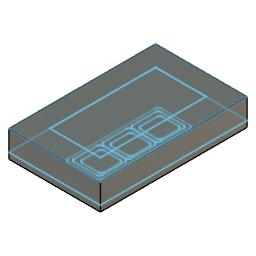
Hackpad (Autodesk Fusion 360 design; units mm, degrees)
part number: 2026-05-27-11-06-18-475
Autodesk Fusion 360 part; units mm, degrees
sketch "Sketch3" plane through (0, 0, 0) normal (0, 1, 0) x (1, 0, 0)
  line L0 (-10, 3.38, 10) -> (14.69, 3.38, 10)
  line L1 (14.69, 3.38, 10) -> (14.69, 3.38, 61.62)
  line L2 (14.69, 3.38, 61.62) -> (-10, 3.38, 61.62)
  line L3 (-10, 3.38, 61.62) -> (-10, 3.38, 10)
  line L4 (-20, 3.38) -> (24.69, 3.38)
  line L5 (24.69, 3.38, 0) -> (24.69, 3.38, 71.62)
  line L6 (24.69, 3.38, 71.62) -> (-20, 3.38, 71.62)
  line L7 (-20, 3.38, 71.62) -> (-20, 3.38, 0)
extrude "Extrude5" add sketch "Sketch3" along normal blind 3 contours L0 L1 L2 L3 in plane through (0, 0, -3.38) normal (0, 0, -1)
extrude "Extrude6" add sketch "Sketch3" along normal blind 10 contours L4 L5 L6 L7 in plane through (0, 0, -3.38) normal (0, 0, -1)
sketch "Sketch5" plane through (0, 0, -13.38) normal (0, 0, -1) x (1, 0, 0)
  line L0 (14.69, -61.62) -> (-10, -61.62)
  line L1 (-10, -61.62) -> (-10, -10)
  line L2 (-10, -10) -> (14.69, -10)
  line L3 (14.69, -10) -> (14.69, -61.62)
  line L4 (-20, -71.62) -> (24.69, -71.62)
  line L5 (24.69, -71.62) -> (24.69, 0)
  line L6 (24.69, 0) -> (-20, 0)
  line L7 (-20, 0) -> (-20, -71.62)
sketch "Sketch7" plane through (0, 0, -13.38) normal (0, 0, -1) x (1, 0, 0)
  line L0 (24.7, -71.6) -> (-20, -71.6)
  line L1 (-20, -71.6) -> (-20, 0)
  line L2 (-20, 0) -> (24.7, 0)
  line L3 (24.7, 0) -> (24.7, -71.6)
  constraint horizontal L0
  constraint vertical L1
  constraint horizontal L2
  constraint vertical L3
extrude "Extrude7" add sketch "Sketch5" along normal blind 3
sketch "keyboard-layout" plane through (0, 0, -16.38) normal (0, 0, -1) x (-1, 0, 0)
  line L0 (-7.433, 41.2046) -> (0.5045, 41.2046)
  line L1 (-8.733, 43.4219) -> (-9.1622, 43.7087)
  line L2 (-9.449, 44.1379) -> (-9.5497, 44.6442)
  line L3 (-8.2268, 43.3212) -> (-8.733, 43.4219)
  line L4 (-9.1622, 43.7087) -> (-9.449, 44.1379)
  line L5 (-8.6552, 40.3879) -> (-8.3685, 40.8171)
  line L6 (4.1079, 44.1379) -> (3.8212, 43.7087)
  line L7 (-8.2268, 43.3212) -> (-8.733, 43.4219)
  line L8 (-9.1622, 43.7087) -> (-9.449, 44.1379)
  line L9 (-8.7559, 46.2317) -> (-8.7559, 54.1691)
  line L10 (-8.7559, 54.1691) -> (-8.6552, 54.6754)
  line L11 (-8.3685, 55.1046) -> (-7.9393, 55.3914)
  line L12 (-9.449, 56.2629) -> (-9.1622, 56.6921)
  line L13 (1.7267, 45.7254) -> (1.4399, 45.2962)
  line L14 (3.8212, 56.6921) -> (4.1079, 56.2629)
  line L15 (3.392, 56.9789) -> (3.8212, 56.6921)
  line L16 (-7.9393, 45.0094) -> (-8.3685, 45.2962)
  line L17 (1.0107, 45.0094) -> (0.5045, 44.9087)
  line L18 (4.2086, 55.7566) -> (4.2086, 44.6442)
  line L19 (-7.433, 55.4921) -> (0.5045, 55.4921)
  line L20 (-8.3685, 55.1046) -> (-7.9393, 55.3914)
  line L21 (-8.7559, 46.2317) -> (-8.7559, 54.1691)
  line L22 (-9.1622, 56.6921) -> (-8.733, 56.9789)
  line L23 (-8.6552, 54.6754) -> (-8.3685, 55.1046)
  line L24 (0.5045, 55.4921) -> (1.0107, 55.3914)
  line L25 (-8.3685, 45.2962) -> (-8.6552, 45.7254)
  line L26 (-8.6552, 45.7254) -> (-8.7559, 46.2317)
  line L27 (2.8857, 43.3212) -> (-8.2268, 43.3212)
  line L28 (2.8857, 57.0796) -> (3.392, 56.9789)
  line L29 (0.5045, 55.4921) -> (1.0107, 55.3914)
  line L30 (1.0107, 55.3914) -> (1.4399, 55.1046)
  line L31 (-7.433, 44.9087) -> (-7.9393, 45.0094)
  line L32 (0.5045, 44.9087) -> (-7.433, 44.9087)
  line L33 (1.4399, 55.1046) -> (1.7267, 54.6754)
  line L34 (-8.733, 43.4219) -> (-9.1622, 43.7087)
  line L35 (-8.6552, 54.6754) -> (-8.3685, 55.1046)
  line L36 (1.8274, 54.1691) -> (1.8274, 46.2317)
  line L37 (3.8212, 43.7087) -> (3.392, 43.4219)
  line L38 (1.4399, 55.1046) -> (1.7267, 54.6754)
  line L39 (1.4399, 45.2962) -> (1.0107, 45.0094)
  line L40 (-9.449, 44.1379) -> (-9.5497, 44.6442)
  line L41 (1.7267, 54.6754) -> (1.8274, 54.1691)
  line L42 (1.8274, 54.1691) -> (1.8274, 46.2317)
  line L43 (1.4399, 45.2962) -> (1.0107, 45.0094)
  line L44 (-7.433, 55.4921) -> (0.5045, 55.4921)
  line L45 (0.5045, 44.9087) -> (-7.433, 44.9087)
  line L46 (-8.733, 56.9789) -> (-8.2268, 57.0796)
  line L47 (1.8274, 46.2317) -> (1.7267, 45.7254)
  line L48 (4.2086, 44.6442) -> (4.1079, 44.1379)
  line L49 (-7.9393, 55.3914) -> (-7.433, 55.4921)
  line L50 (4.1079, 56.2629) -> (4.2086, 55.7566)
  line L51 (-8.2268, 57.0796) -> (2.8857, 57.0796)
  line L52 (1.0107, 45.0094) -> (0.5045, 44.9087)
  line L53 (1.8274, 46.2317) -> (1.7267, 45.7254)
  line L54 (1.7267, 45.7254) -> (1.4399, 45.2962)
  line L55 (-7.433, 44.9087) -> (-7.9393, 45.0094)
  line L56 (-8.7559, 54.1691) -> (-8.6552, 54.6754)
  line L57 (-7.9393, 45.0094) -> (-8.3685, 45.2962)
  line L58 (1.0107, 55.3914) -> (1.4399, 55.1046)
  line L59 (-7.9393, 55.3914) -> (-7.433, 55.4921)
  line L60 (-8.3685, 45.2962) -> (-8.6552, 45.7254)
  line L61 (3.392, 43.4219) -> (2.8857, 43.3212)
  line L62 (-9.5497, 44.6442) -> (-9.5497, 55.7566)
  line L63 (-8.6552, 45.7254) -> (-8.7559, 46.2317)
  line L64 (1.7267, 54.6754) -> (1.8274, 54.1691)
  line L65 (2.8857, 42.7921) -> (3.392, 42.6914)
  line L66 (-8.6552, 17.1504) -> (-8.7559, 17.6567)
  line L67 (-7.9393, 26.8164) -> (-7.433, 26.9171)
  line L68 (2.8857, 42.7921) -> (3.392, 42.6914)
  line L69 (3.8212, 29.4212) -> (3.392, 29.1345)
  line L70 (-9.5497, 55.7566) -> (-9.449, 56.2629)
  line L71 (1.4399, 16.7212) -> (1.0107, 16.4345)
  line L72 (3.392, 29.1345) -> (2.8857, 29.0338)
  line L73 (-8.6552, 17.1504) -> (-8.7559, 17.6567)
  line L74 (-9.5497, 41.4692) -> (-9.449, 41.9754)
  line L75 (-7.433, 16.3338) -> (-7.9393, 16.4345)
  line L76 (0.5045, 16.3338) -> (-7.433, 16.3338)
  line L77 (1.8274, 17.6567) -> (1.7267, 17.1504)
  line L78 (-7.9393, 16.4345) -> (-8.3685, 16.7212)
  line L79 (-8.3685, 16.7212) -> (-8.6552, 17.1504)
  line L80 (-8.2268, 42.7921) -> (2.8857, 42.7921)
  line L81 (-7.9393, 16.4345) -> (-8.3685, 16.7212)
  line L82 (1.7267, 26.1004) -> (1.8274, 25.5942)
  line L83 (1.0107, 16.4345) -> (0.5045, 16.3338)
  line L84 (4.2086, 41.4692) -> (4.2086, 30.3567)
  line L85 (-9.1622, 29.4212) -> (-9.449, 29.8504)
  line L86 (-8.733, 42.6914) -> (-8.2268, 42.7921)
  line L87 (3.392, 42.6914) -> (3.8212, 42.4046)
  line L88 (4.1079, 29.8504) -> (3.8212, 29.4212)
  line L89 (-8.733, 29.1345) -> (-9.1622, 29.4212)
  line L90 (-8.2268, 42.7921) -> (2.8857, 42.7921)
  line L91 (1.8274, 25.5942) -> (1.8274, 17.6567)
  line L92 (4.1079, 29.8504) -> (3.8212, 29.4212)
  line L93 (-8.3685, 16.7212) -> (-8.6552, 17.1504)
  line L94 (-9.449, 29.8504) -> (-9.5497, 30.3567)
  line L95 (-9.5497, 41.4692) -> (-9.449, 41.9754)
  line L96 (4.2086, 41.4692) -> (4.2086, 30.3567)
  line L97 (4.2086, 30.3567) -> (4.1079, 29.8504)
  line L98 (4.1079, 41.9754) -> (4.2086, 41.4692)
  line L99 (0.5045, 26.9171) -> (1.0107, 26.8164)
  line L100 (3.8212, 42.4046) -> (4.1079, 41.9754)
  line L101 (4.2086, 30.3567) -> (4.1079, 29.8504)
  line L102 (1.4399, 26.5296) -> (1.7267, 26.1004)
  line L103 (-8.7559, 17.6567) -> (-8.7559, 25.5942)
  line L104 (2.8857, 29.0338) -> (-8.2268, 29.0338)
  line L105 (-9.5497, 30.3567) -> (-9.5497, 41.4692)
  line L106 (-9.1622, 42.4046) -> (-8.733, 42.6914)
  line L107 (-8.7559, 25.5942) -> (-8.6552, 26.1004)
  line L108 (-8.2268, 29.0338) -> (-8.733, 29.1345)
  line L109 (1.0107, 41.1039) -> (1.4399, 40.8171)
  line L110 (0.5045, 30.6213) -> (-7.433, 30.6213)
  line L111 (1.7267, 40.3879) -> (1.8274, 39.8817)
  line L112 (1.4399, 31.0087) -> (1.0107, 30.722)
  line L113 (-8.6552, 31.4379) -> (-8.7559, 31.9442)
  line L114 (0.5045, 41.2046) -> (1.0107, 41.1039)
  line L115 (-8.2268, 29.0338) -> (-8.733, 29.1345)
  line L116 (1.8274, 31.9442) -> (1.7267, 31.4379)
  line L117 (-8.3685, 40.8171) -> (-7.9393, 41.1039)
  line L118 (1.8274, 31.9442) -> (1.7267, 31.4379)
  line L119 (-7.9393, 41.1039) -> (-7.433, 41.2046)
  line L120 (1.7267, 40.3879) -> (1.8274, 39.8817)
  line L121 (-8.6552, 31.4379) -> (-8.7559, 31.9442)
  line L122 (-9.5497, 55.7566) -> (-9.449, 56.2629)
  line L123 (0.5045, 30.6213) -> (-7.433, 30.6213)
  line L124 (0.5045, 41.2046) -> (1.0107, 41.1039)
  line L125 (1.4399, 31.0087) -> (1.0107, 30.722)
  line L126 (1.0107, 30.722) -> (0.5045, 30.6213)
  line L127 (-7.433, 41.2046) -> (0.5045, 41.2046)
  line L128 (-7.433, 30.6213) -> (-7.9393, 30.722)
  line L129 (-8.7559, 39.8817) -> (-8.6552, 40.3879)
  line L130 (-8.7559, 39.8817) -> (-8.6552, 40.3879)
  line L131 (-8.7559, 31.9442) -> (-8.7559, 39.8817)
  line L132 (-7.9393, 41.1039) -> (-7.433, 41.2046)
  line L133 (1.8274, 39.8817) -> (1.8274, 31.9442)
  line L134 (-8.3685, 31.0087) -> (-8.6552, 31.4379)
  line L135 (-8.7559, 31.9442) -> (-8.7559, 39.8817)
  line L136 (-9.5497, 44.6442) -> (-9.5497, 55.7566)
  line L137 (-8.2268, 57.0796) -> (2.8857, 57.0796)
  line L138 (1.4399, 40.8171) -> (1.7267, 40.3879)
  line L139 (1.8274, 39.8817) -> (1.8274, 31.9442)
  line L140 (1.7267, 31.4379) -> (1.4399, 31.0087)
  line L141 (-8.733, 56.9789) -> (-8.2268, 57.0796)
  line L142 (2.8857, 57.0796) -> (3.392, 56.9789)
  line L143 (1.4399, 40.8171) -> (1.7267, 40.3879)
  line L144 (-9.1622, 56.6921) -> (-8.733, 56.9789)
  line L145 (-7.433, 30.6213) -> (-7.9393, 30.722)
  line L146 (3.392, 56.9789) -> (3.8212, 56.6921)
  line L147 (3.8212, 56.6921) -> (4.1079, 56.2629)
  line L148 (-7.9393, 30.722) -> (-8.3685, 31.0087)
  line L149 (-9.1622, 29.4212) -> (-9.449, 29.8504)
  line L150 (4.1079, 56.2629) -> (4.2086, 55.7566)
  line L151 (-8.6552, 40.3879) -> (-8.3685, 40.8171)
  line L152 (-8.3685, 31.0087) -> (-8.6552, 31.4379)
  line L153 (4.2086, 44.6442) -> (4.1079, 44.1379)
  line L154 (-9.449, 56.2629) -> (-9.1622, 56.6921)
  line L155 (3.392, 43.4219) -> (2.8857, 43.3212)
  line L156 (4.1079, 44.1379) -> (3.8212, 43.7087)
  line L157 (3.8212, 43.7087) -> (3.392, 43.4219)
  line L158 (2.8857, 43.3212) -> (-8.2268, 43.3212)
  line L159 (2.8857, 29.0338) -> (-8.2268, 29.0338)
  line L160 (1.0107, 41.1039) -> (1.4399, 40.8171)
  line L161 (1.0107, 30.722) -> (0.5045, 30.6213)
  line L162 (4.2086, 55.7566) -> (4.2086, 44.6442)
  line L163 (-11.1372, 14.7463) -> (-11.1372, 57.0795)
  line L164 (4.1079, 15.5629) -> (3.8212, 15.1337)
  line L165 (3.392, 14.847) -> (2.8857, 14.7463)
  line L166 (4.2086, 27.1817) -> (4.2086, 16.0692)
  line L167 (-11.0124, 57.6975) -> (-10.6722, 58.2021)
  line L168 (4.2086, 58.667) -> (4.8266, 58.5423)
  line L169 (-11.1372, 57.0795) -> (-11.0124, 57.6975)
  line L170 (-9.449, 29.8504) -> (-9.5497, 30.3567)
  line L171 (-7.9393, 30.722) -> (-8.3685, 31.0087)
  line L172 (-8.733, 29.1345) -> (-9.1622, 29.4212)
  line L173 (-10.1676, 58.5423) -> (-9.5497, 58.667)
  line L174 (-9.5497, 58.667) -> (4.2086, 58.667)
  line L175 (5.3312, 58.2021) -> (5.6714, 57.6975)
  line L176 (5.6714, 57.6975) -> (5.7961, 57.0795)
  line L177 (5.7961, 57.0795) -> (5.7961, 14.7463)
  line L178 (-10.6722, 13.6237) -> (-11.0163, 14.1388)
  line L179 (-8.3685, 40.8171) -> (-7.9393, 41.1039)
  line L180 (4.8266, 58.5423) -> (5.3312, 58.2021)
  line L181 (-10.6722, 58.2021) -> (-10.1676, 58.5423)
  line L182 (-9.5497, 13.1588) -> (-10.1572, 13.2796)
  line L183 (-8.2268, 28.5046) -> (2.8857, 28.5046)
  line L184 (2.8857, 28.5046) -> (3.392, 28.4039)
  line L185 (1.7267, 31.4379) -> (1.4399, 31.0087)
  line L186 (5.3312, 13.6237) -> (4.8162, 13.2796)
  line L187 (-9.1622, 28.1171) -> (-8.733, 28.4039)
  line L188 (-11.0163, 14.1388) -> (-11.1372, 14.7463)
  line L189 (-8.733, 28.4039) -> (-8.2268, 28.5046)
  line L190 (4.2086, 13.1588) -> (-9.5497, 13.1588)
  line L191 (3.392, 28.4039) -> (3.8212, 28.1171)
  line L192 (5.6753, 14.1388) -> (5.3312, 13.6237)
  line L193 (-8.2268, 14.7463) -> (-8.733, 14.847)
  line L194 (3.8212, 15.1337) -> (3.392, 14.847)
  line L195 (-9.5497, 16.0692) -> (-9.5497, 27.1817)
  line L196 (-10.1572, 13.2796) -> (-10.6722, 13.6237)
  line L197 (4.1079, 27.6879) -> (4.2086, 27.1817)
  line L198 (-9.449, 27.6879) -> (-9.1622, 28.1171)
  line L199 (-9.5497, 27.1817) -> (-9.449, 27.6879)
  line L200 (3.8212, 28.1171) -> (4.1079, 27.6879)
  line L201 (2.8857, 14.7463) -> (-8.2268, 14.7463)
  line L202 (5.7961, 14.7463) -> (5.6753, 14.1388)
  line L203 (4.8162, 13.2796) -> (4.2086, 13.1588)
  line L204 (4.2086, 16.0692) -> (4.1079, 15.5629)
  line L205 (-8.733, 14.847) -> (-9.1622, 15.1337)
  line L206 (-9.1622, 15.1337) -> (-9.449, 15.5629)
  line L207 (-9.449, 15.5629) -> (-9.5497, 16.0692)
  line L208 (-9.5497, 16.0692) -> (-9.5497, 27.1817)
  line L209 (-9.449, 27.6879) -> (-9.1622, 28.1171)
  line L210 (-9.5497, 27.1817) -> (-9.449, 27.6879)
  line L211 (-8.2268, 28.5046) -> (2.8857, 28.5046)
  line L212 (-9.1622, 28.1171) -> (-8.733, 28.4039)
  line L213 (-8.733, 28.4039) -> (-8.2268, 28.5046)
  line L214 (2.8857, 28.5046) -> (3.392, 28.4039)
  line L215 (3.392, 28.4039) -> (3.8212, 28.1171)
  line L216 (3.8212, 28.1171) -> (4.1079, 27.6879)
  line L217 (4.1079, 27.6879) -> (4.2086, 27.1817)
  line L218 (4.2086, 27.1817) -> (4.2086, 16.0692)
  line L219 (-8.2268, 14.7463) -> (-8.733, 14.847)
  line L220 (-9.449, 15.5629) -> (-9.5497, 16.0692)
  line L221 (4.1079, 15.5629) -> (3.8212, 15.1337)
  line L222 (-8.3685, 26.5296) -> (-7.9393, 26.8164)
  line L223 (1.4399, 26.5296) -> (1.7267, 26.1004)
  line L224 (-7.433, 16.3338) -> (-7.9393, 16.4345)
  line L225 (-7.433, 26.9171) -> (0.5045, 26.9171)
  line L226 (-8.733, 14.847) -> (-9.1622, 15.1337)
  line L227 (-7.9393, 26.8164) -> (-7.433, 26.9171)
  line L228 (-8.6552, 26.1004) -> (-8.3685, 26.5296)
  line L229 (1.7267, 26.1004) -> (1.8274, 25.5942)
  line L230 (-9.449, 41.9754) -> (-9.1622, 42.4046)
  line L231 (-9.1622, 42.4046) -> (-8.733, 42.6914)
  line L232 (4.2086, 16.0692) -> (4.1079, 15.5629)
  line L233 (-7.433, 26.9171) -> (0.5045, 26.9171)
  line L234 (1.0107, 16.4345) -> (0.5045, 16.3338)
  line L235 (-9.1622, 15.1337) -> (-9.449, 15.5629)
  line L236 (0.5045, 26.9171) -> (1.0107, 26.8164)
  line L237 (-9.5497, 30.3567) -> (-9.5497, 41.4692)
  line L238 (1.8274, 25.5942) -> (1.8274, 17.6567)
  line L239 (1.7267, 17.1504) -> (1.4399, 16.7212)
  line L240 (0.5045, 16.3338) -> (-7.433, 16.3338)
  line L241 (1.0107, 26.8164) -> (1.4399, 26.5296)
  line L242 (-8.7559, 25.5942) -> (-8.6552, 26.1004)
  line L243 (3.392, 42.6914) -> (3.8212, 42.4046)
  line L244 (-9.449, 41.9754) -> (-9.1622, 42.4046)
  line L245 (1.4399, 16.7212) -> (1.0107, 16.4345)
  line L246 (-8.6552, 26.1004) -> (-8.3685, 26.5296)
  line L247 (3.392, 14.847) -> (2.8857, 14.7463)
  line L248 (2.8857, 14.7463) -> (-8.2268, 14.7463)
  line L249 (-8.3685, 26.5296) -> (-7.9393, 26.8164)
  line L250 (-8.733, 42.6914) -> (-8.2268, 42.7921)
  line L251 (-8.7559, 17.6567) -> (-8.7559, 25.5942)
  line L252 (1.7267, 17.1504) -> (1.4399, 16.7212)
  line L253 (3.8212, 42.4046) -> (4.1079, 41.9754)
  line L254 (3.8212, 15.1337) -> (3.392, 14.847)
  line L255 (1.8274, 17.6567) -> (1.7267, 17.1504)
  line L256 (3.8212, 29.4212) -> (3.392, 29.1345)
  line L257 (4.1079, 41.9754) -> (4.2086, 41.4692)
  line L258 (3.392, 29.1345) -> (2.8857, 29.0338)
  line L259 (1.0107, 26.8164) -> (1.4399, 26.5296)
